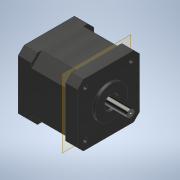
# Autodesk Inventor part: Шаговик17
Saved by Autodesk Inventor 2020 (Build 240168000, 168)
## iProperties
Created: 2021-03-14
Part Number: Шаговик17
Material: Сталь, литейная
Document SubType Name: Modeling
Designer: I_Love_U_Bogdan
Density: 7.85 g/cm^3
Appearance: Темно-серый
Author: I_Love_U_Bogdan
Autodesk Inventor part; units mm, degrees
ref_plane "YZ Plane" through (0, 0, 0) normal (1, 0, 0) x (0, 1, 0)
ref_plane "XZ Plane" through (0, 0, 0) normal (0, 1, 0) x (-1, 0, 0)
ref_plane "XY Plane" through (0, 0, 0) normal (0, 0, 1) x (1, 0, 0)
sketch "Эскиз1" plane through (0, 0, 0) normal (1, 0, 0) x (0, 1, 0)
  line L0 (-17, 21) -> (17, 21)
  line L1 (21, 17) -> (21, -17)
  line L2 (17, -21) -> (-17, -21)
  line L3 (-21, -17) -> (-21, 17)
  line L4 (-21, 21) -> (21, -21) construction
  line L5 (21, 21) -> (-21, -21) construction
  line L6 (21, 17) -> (17, 21)
  line L7 (21, -17) -> (17, -21)
  line L8 (-17, 21) -> (-21, 17)
  line L9 (-21, -17) -> (-17, -21)
  point P0 (0, 0)
  dimension "d0" = 42
  dimension "d1" = 42
  dimension "d2" = 4
  dimension "d3" = 4
  dimension "d4" = 4
  dimension "d5" = 4
  dimension "d6" = 4
  dimension "d7" = 4
  dimension "d8" = 4
  dimension "d9" = 4
  constraints: 20 end point, 8 point on line, 2 midpoint, 2 parallel, 1 horizontal, 1 perpendicular
  measures "d0" distance of L4.end L5.end
  measures "d1" distance of L5.start L4.end
  measures "d2" distance of L1.start L5.start
  measures "d3" distance of L0.end L5.start
  measures "d4" distance of L1.end L4.end
  measures "d5" distance of L2.start L4.end
  measures "d6" distance of L0.start L4.start
  measures "d7" distance of L3.end L4.start
  measures "d8" distance of L3.start L5.end
  measures "d9" distance of L2.end L5.end
extrude "Выдавливание1" add sketch "Эскиз1" against normal blind 40
ref_plane "РабПлоскость1" through (-8, 0, 0) normal (1, 0, 0) x (0, 0, -1)
sketch "Эскиз2" plane through (-8, 0, 0) normal (1, 0, 0) x (0, 0, -1)
  line L0 (-21, -17) -> (-17, -21)
  line L1 (-14, -21) -> (14, -21)
  line L2 (17, -21) -> (21, -17)
  line L3 (21, -14) -> (21, 14)
  line L4 (21, 17) -> (17, 21)
  line L5 (17, 21) -> (-14, 21)
  line L6 (-17, 21) -> (-21, 17)
  line L7 (-21, 14) -> (-21, -14)
  line L8 (14, 21) -> (-17, 21)
  line L9 (-21, -17) -> (-21, 17)
  line L10 (21, -17) -> (21, 17)
  line L11 (-17, -21) -> (17, -21)
  line L12 (-14, 21) -> (-21, 14)
  line L13 (-21, -14) -> (-14, -21)
  line L14 (21, -14) -> (14, -21)
  line L15 (21, 14) -> (14, 21)
  point P0 (0, 0)
  point P1 (-21, 21)
  point P2 (-21, -21)
  point P3 (21, -21)
  point P4 (21, 21)
  point P5 (14, -21)
  point P6 (-14, 21)
  dimension "d14" = 7
  dimension "d15" = 7
  dimension "d16" = 7
  dimension "d17" = 7
  dimension "d18" = 7
  dimension "d19" = 7
  dimension "d20" = 7
  dimension "d21" = 7
  constraints: 32 end point, 16 point on line
  measures "d14" distance of L5.end point (-21, 21)
  measures "d15" distance of L7.start point (-21, 21)
  measures "d16" distance of L7.end point (-21, -21)
  measures "d17" distance of L1.start point (-21, -21)
  measures "d18" distance of L3.start point (21, -21)
  measures "d19" distance of L1.end point (21, -21)
  measures "d20" distance of L3.end point (21, 21)
  measures "d21" distance of L8.start point (21, 21)
extrude "Выдавливание2" cut sketch "Эскиз2" against normal blind 23 contours L9 L13 L11 L0 | L9 L6 L8 L12 | L14 L10 L2 L11 | L5 L4 L10 L15
sketch "Эскиз3" plane through (0, 0, 0) normal (1, 0, 0) x (0, 0, -1)
  line L0 (-21, -17) -> (-17, -21) projected
  line L1 (-17, -21) -> (17, -21) projected
  line L2 (17, -21) -> (21, -17) projected
  line L3 (21, -17) -> (21, 17) projected
  line L4 (21, 17) -> (17, 21) projected
  line L5 (17, 21) -> (-17, 21) projected
  line L6 (-17, 21) -> (-21, 17) projected
  line L7 (-21, 17) -> (-21, -17) projected
  circle A0 centre (0, 0) radius 2.5
  dimension "d24" = 5
  constraints: 1 centre point, 1 coincident
  measures "d24" diameter of A0
extrude "Выдавливание3" add sketch "Эскиз3" along normal blind 15 contours A0
sketch "Эскиз4" plane through (0, 0, 0) normal (1, 0, 0) x (0, 0, -1)
  line L0 (-15.5, -15.5) -> (15.5, -15.5)
  line L1 (15.5, -15.5) -> (15.5, 15.5)
  line L2 (15.5, 15.5) -> (-15.5, 15.5)
  line L3 (-15.5, 15.5) -> (-15.5, -15.5)
  line L4 (-15.5, -15.5) -> (15.5, 15.5) construction
  line L5 (15.5, -15.5) -> (-15.5, 15.5) construction
  circle A0 centre (-15.5, 15.5) radius 1.5
  circle A1 centre (15.5, 15.5) radius 1.5
  circle A2 centre (15.5, -15.5) radius 1.5
  circle A3 centre (-15.5, -15.5) radius 1.5
  point P0 (0, 0)
  dimension "d27" = 31
  dimension "d28" = 31
  dimension "d29" = 3
  dimension "d30" = 3
  dimension "d31" = 3
  dimension "d32" = 3
  constraints: 12 end point, 4 centre point, 3 coincident, 2 midpoint, 2 parallel, 1 horizontal, 1 perpendicular
  measures "d27" distance of L2.end L1.end
  measures "d28" distance of L1.end L0.end
  measures "d29" diameter of A0
  measures "d30" diameter of A1
  measures "d31" diameter of A2
  measures "d32" diameter of A3
extrude "Выдавливание4" cut sketch "Эскиз4" against normal blind 8 contours L3 A3 L0 | L0 A3 L3 | A2 L1 L0 | L0 L1 A2 | A0 L2 L3 | L3 L2 A0 | A1 L2 L1 | L1 L2 A1
sketch "Эскиз5" plane through (15, 0, 0) normal (1, 0, 0) x (0, 0, -1)
  point P0 (0, 0)
sketch "Эскиз6" plane through (0, 0, 0) normal (1, 0, 0) x (0, 0, -1)
  circle A0 centre (0, 0) radius 2.5 projected
  circle A1 centre (0, 0) radius 11
  circle A2 centre (0, 0) radius 5
  dimension "d35" = 22
  dimension "d36" = 6
  constraints: 2 centre point, 1 coincident
  measures "d35" diameter of A1
  measures "d36" radial gap between concentric circles of A1 A2
extrude "Выдавливание5" add sketch "Эскиз6" along normal blind 2 contours A1
equation "\"d3\" = d2"
equation "\"d4\" = d2"
equation "\"d5\" = d4"
equation "\"d6\" = d2"
equation "\"d7\" = d6"
equation "\"d8\" = d2"
equation "\"d9\" = d8"
equation "\"d15\" = d14"
equation "\"d16\" = d14"
equation "\"d17\" = d16"
equation "\"d18\" = d14"
equation "\"d19\" = d18"
equation "\"d20\" = d14"
equation "\"d21\" = d20"
